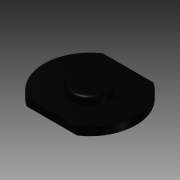
# Autodesk Inventor part: plaque moteur
Saved by Autodesk Inventor 2014 SP2 (Build 180246200, 246)
## iProperties
Created: 2015-03-17
Part Number: plaque moteur
Material: Résine acétal, noir
Document SubType Name: Modeling
Designer: sd
Density: 1.425 g/cm^3
Appearance: Lisse - Noir
Mass: 0.17588 g
Surface Area: 2.58687 cm^2
Volume: 0.123424 cm^3
Author: sd
Autodesk Inventor part; units mm, degrees
ref_plane "YZ Plane" through (0, 0, 0) normal (1, 0, 0) x (0, 1, 0)
ref_plane "XZ Plane" through (0, 0, 0) normal (0, 1, 0) x (-1, 0, 0)
ref_plane "XY Plane" through (0, 0, 0) normal (0, 0, 1) x (1, 0, 0)
sketch "Esquisse1" plane through (0, 0, 0) normal (0, 0, 1) x (1, 0, 0)
  circle A0 centre (0, 0) radius 6
  line L0 (-3.3166, 5) -> (3.3166, 5)
  line L1 (-3.3166, -5) -> (3.3166, -5)
  dimension "d0" = 12
  dimension "d1" = 10
  dimension "d2" = 5
  constraints: 4 end point, 4 point on circle, 1 centre point, 1 coincident, 1 horizontal, 1 parallel
  measures "d0" diameter of A0
  measures "d1" distance between parallel lines of L1 L0
  measures "d2" distance from line of point (0, 0) L0
extrude "Extrusion1" add sketch "Esquisse1" along normal blind 1 contours A0 L1 L0
fillet "Congé1" radius 0.5 4 edges at (-3.3166, 5, 0.5) (3.3166, 5, 0.5) (-3.3166, -5, 0.5) (3.3166, -5, 0.5)
sketch "Esquisse2" plane through (0, 0, 1) normal (0, 0, 1) x (1, 0, 0)
  arc A0 (-3.4498, 4.9091) -> (-3.4498, -4.9091) centre (0, 0) ccw projected
  circle A1 centre (0, 0) radius 2.5
  dimension "d6" = 5
  constraints: 1 centre point, 1 coincident
  measures "d6" diameter of A1
extrude "Extrusion2" add sketch "Esquisse2" along normal blind 1
fillet "Congé2" radius 0.3 1 edges at (-2.5, 0, 2)
equation "\"d2\" = 0.5 * d1"
